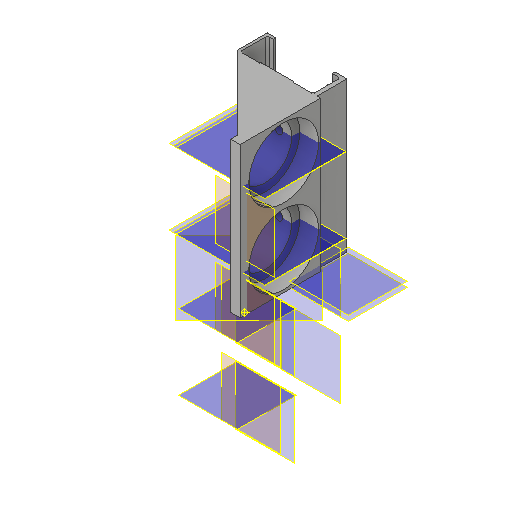
# Autodesk Inventor part: 30_Cube_Insert_Filter_Revolver_Filter_base_triple
Saved by Autodesk Inventor 2022 (Build 260153000, 153)
## iProperties
Created: 2021-09-13
Part Number: 30_Cube_Insert_Filter_Revolver_Filter_base_triple
Material: Generic
Document SubType Name: Modeling
Designer: diederichbenedict
Density: 1 g/cm^3
Appearance: Default
Mass: 6.97028 g
Surface Area: 48.8121 cm^2
Volume: 6.97028 cm^3
Author: diederichbenedict
Autodesk Inventor part; units mm, degrees
ref_plane "YZ Plane" through (0, 0, 0) normal (1, 0, 0) x (0, 1, 0)
ref_plane "XZ Plane" through (0, 0, 0) normal (0, 1, 0) x (-1, 0, 0)
ref_plane "XY Plane" through (0, 0, 0) normal (0, 0, 1) x (1, 0, 0)
ref_plane "Work Plane1" through (-34.3358, -34.38, 2.0699) normal (0, -1, 0) x (0.7071068, 0, -0.7071068)
ref_plane "Work Plane4" through (-9.5871, -34.38, 28.2329) normal (0, -1, 0) x (1, 0, 0)
ref_plane "Work Plane3" through (-9.5871, -32.38, 28.2329) normal (0, -1, 0) x (1, 0, 0)
sketch "Sketch1" plane through (-9.5871, -34.38, 28.2329) normal (0, -1, 0) x (1, 0, 0)
  line L0 (0.7071, -1.3185) -> (0.7071, -26.3185) construction
  line L1 (0.7071, -1.3185) -> (1.7071, -1.3185) construction
  line L2 (0.7071, -26.3185) -> (1.7071, -26.3185) construction
  line L3 (-4.2929, -0.7071) -> (-31.7929, -28.2071)
  line L4 (-31.7929, -28.2071) -> (0.7071, -28.2071)
  line L5 (0.7071, -28.2071) -> (0.7071, -0.7071)
  line L6 (0.7071, -0.7071) -> (-4.2929, -0.7071)
  line L7 (-4.2929, -0.7071) -> (-4.2929, -28.2071)
  line L8 (-4.2929, -28.2071) -> (0.7071, -28.2071)
  line L9 (0.7071, -0.7071) -> (3.5978, -0.7071)
  line L10 (2.5336, 1.8671) -> (2.3871, 1.8671) projected
  line L11 (0.7071, -0.7071) -> (0.7071, -28.2071)
  line L12 (0.7071, -28.2071) -> (-31.7929, -28.2071)
  point P0 (9.5871, -28.2329)
  dimension "d1" = 5
  dimension "d96" = 27.5
  dimension "d97" = 135
  constraints: 22 end point, 4 perpendicular, 3 horizontal, 2 point on line, 1 collinear, 2 other
  measures "d1" distance of L5.end L3.start
  measures "d96" distance between parallel lines of L4 L6
  measures "d97" angle of L7 L3
extrude "Extrusion1" add sketch "Sketch1" against normal blind 28
ref_plane "Work Plane5" through (-9.5871, -20.38, 28.2329) normal (0, -1, 0) x (1, 0, 0)
ref_plane "Work Plane6" through (-11.0013, -34.38, 27.5258) normal (0, 0, 1) x (1, 0, 0)
sketch "Sketch4" plane through (-8.88, -34.38, 27.5258) normal (-1, 0, 0) x (0, 0, 1)
  line L0 (0, 0) -> (-27.5, 0) projected
  line L1 (-27.5, 28) -> (0, 28) projected
  circle A0 centre (-13.75, 14) radius 10
  line L2 (0, 0) -> (0, 28) projected
  point P0 (-27.5258, 34.38)
  dimension "d89" = 28
  dimension "d90" = 20
  dimension "d91" = 14
  dimension "d98" = 13.75
  constraints: 1 centre point
  measures "d89" distance between parallel lines of L0 L1
  measures "d90" diameter of A0
  measures "d91" distance from line of A0.centre L0
  measures "d98" distance from line of A0.centre L2
extrude "Extrusion4" cut sketch "Sketch4" along normal through all
sketch "Sketch9" plane through (-11.38, -34.38, 30.0258) normal (-0.7071068, 0, 0.7071068) x (0.7071068, 0, 0.7071068)
  ellipse E0 centre (-22.981, 14) end of major axis (-37.1231, 14) minor radius 10 projected
  circle A0 centre (-22.981, 14) radius 13
  point P0 (-13.1846, 34.38)
  dimension "d129" = 26
  constraints: 1 centre point, 1 coincident, 1 other
  measures "d129" diameter of A0
extrude "Extrusion9" cut sketch "Sketch9" against normal blind 3.3 contours A0 E0 | E0 A0 | A0 E0 picked at (-32.6632, 13.9035) picked at (-21.8913, 2.1109) picked at (-24.0707, 25.8891)
sketch "Sketch3" plane through (-8.88, -34.38, 27.5258) normal (-1, 0, 0) x (0, 0, 1)
  circle A0 centre (-13.75, 14) radius 10 projected
  circle A1 centre (-13.75, 14) radius 13
  point P0 (-27.5258, 34.38)
  point P1 (13.1114, 14)
  dimension "d100" = 26
  constraints: 1 centre point, 1 coincident
  measures "d100" diameter of A1
extrude "Extrusion3" cut sketch "Sketch3" along normal blind 8.5 contours A0 | A1
sketch "Sketch13" plane through (-12.38, -34.38, 29.0258) normal (-0.7071068, 0, 0.7071068) x (0.7071068, 0, 0.7071068)
  arc A0 (-7.4246, 14) -> (-7.4246, 14) centre (-21.5668, 14) ccw projected
  circle A1 centre (-7.0668, 25) radius 1.4
  circle A2 centre (-7.0668, 3) radius 1.4
  circle A3 centre (-37.5668, 14) radius 1.4
  point P0 (-11.7703, 34.38)
  point P1 (-18.5424, 14)
  dimension "d101" = 2.8
  dimension "d102" = 2.8
  dimension "d103" = 14.5
  dimension "d104" = 14.5
  dimension "d105" = 16
  dimension "d106" = 2.8
  dimension "d127" = 11
  dimension "d128" = 11
  constraints: 3 centre point, 1 other
  measures "d101" diameter of A2
  measures "d102" diameter of A3
  measures "d103" horizontal distance of A1.centre point (-21.567, 14)
  measures "d104" horizontal distance of point (-21.567, 14) A2.centre
  measures "d105" distance of point (-21.567, 14) A3.centre
  measures "d106" diameter of A1
  measures "d127" vertical distance of A1.centre point (-21.567, 14)
  measures "d128" vertical distance of point (-21.567, 14) A2.centre
extrude "Extrusion13" cut sketch "Sketch13" against normal blind 10 contours A1 | A2 | A3
ref_plane "Arbeitsebene13" through (-3.6065, -62.7242, 27.5258) normal (0, 0, -1) x (-1, 0, 0)
ref_plane "Arbeitsebene16" through (-8.88, -62.38, 27.5258) normal (0, 0, 1) x (1, 0, 0)
sketch "Sketch16" plane through (-8.88, -62.38, 27.5258) normal (0, 0, 1) x (1, 0, 0)
  ellipse E0 centre (-13.3299, 42) end of major axis (-13.3299, 54.75) minor radius 9.0156 projected
  circle A0 centre (-13.3299, 42) radius 1.5708
  point P0 (8.88, 62.38)
  constraints: 1 centre point, 1 coincident, 1 other
extrude "Extrusion15" cut sketch "Sketch16" against normal through all contours A0
ref_plane "Work Plane11" through (-8.88, -20.38, 27.5258) normal (0, -1, 0) x (1, 0, 0)
ref_plane "Arbeitsebene12" through (-8.88, -20.38, 27.5258) normal (0, -1, 0) x (1, 0, 0)
ref_plane "Arbeitsebene15" through (-13.88, -62.38, 0.0258) normal (0, 0, -1) x (1, 0, 0)
sketch "Skizze20" plane through (-13.88, -62.38, 0.0258) normal (0, 0, -1) x (1, 0, 0)
  circle A0 centre (27.7649, 33.0797) radius 1.45
  point P0 (13.88, -62.38)
  dimension "d93" = 2.9
  constraints: 1 centre point
  measures "d93" diameter of A0
extrude "Extrusion17" cut sketch "Skizze20" against normal blind 10
ref_plane "Arbeitsebene14" through (-13.88, -62.38, 27.5258) normal (0, -1, 0) x (1, 0, 0)
sketch "Skizze22" plane through (-13.88, -34.38, 27.5258) normal (0, -1, 0) x (1, 0, 0)
  arc A0 (-18.7505, -36.1766) -> (-18.1728, -35.6773) centre (-19.2056, -35.0662) ccw projected
  arc A1 (-17.9795, -35.5555) -> (-18.1728, -35.6773) centre (-17.9577, -35.8046) ccw projected
  line L0 (-17.9795, -35.5555) -> (-17.6339, -35.5253) projected
  arc A2 (-17.6339, -35.5253) -> (-17.4056, -35.2762) centre (-17.6556, -35.2762) ccw projected
  line L1 (-17.4056, -35.2762) -> (-17.4056, -34.8238) projected
  arc A3 (-17.4056, -34.8238) -> (-17.6339, -34.5747) centre (-17.6556, -34.8238) ccw projected
  line L2 (-17.6339, -34.5747) -> (-18.0004, -34.5427) projected
  arc A4 (-18.1902, -34.4268) -> (-18.0004, -34.5427) centre (-17.9786, -34.2936) ccw projected
  arc A5 (-18.1902, -34.4268) -> (-18.7505, -33.9559) centre (-19.2056, -35.0662) ccw projected
  arc A6 (-18.9056, -33.7246) -> (-18.7505, -33.9559) centre (-18.6556, -33.7246) ccw projected
  line L3 (-18.9056, -33.7246) -> (-18.9056, -33.05) projected
  line L4 (-18.9056, -33.05) -> (-18.4056, -32.55) projected
  line L5 (-18.4056, -32.55) -> (-7.4056, -32.55) projected
  line L6 (-7.4056, -32.55) -> (-6.9056, -33.05) projected
  line L7 (-6.9056, -33.05) -> (-6.9056, -33.7246) projected
  arc A7 (-7.0608, -33.9559) -> (-6.9056, -33.7246) centre (-7.1556, -33.7246) ccw projected
  arc A8 (-7.0608, -33.9559) -> (-7.6211, -34.4268) centre (-6.6057, -35.0662) ccw projected
  arc A9 (-7.8109, -34.5427) -> (-7.6211, -34.4268) centre (-7.8327, -34.2936) ccw projected
  line L8 (-7.8109, -34.5427) -> (-8.1774, -34.5747) projected
  arc A10 (-8.1774, -34.5747) -> (-8.4056, -34.8238) centre (-8.1556, -34.8238) ccw projected
  line L9 (-8.4056, -34.8238) -> (-8.4056, -35.2762) projected
  arc A11 (-8.4056, -35.2762) -> (-8.1774, -35.5253) centre (-8.1556, -35.2762) ccw projected
  line L10 (-8.1774, -35.5253) -> (-7.8318, -35.5555) projected
  arc A12 (-7.6384, -35.6773) -> (-7.8318, -35.5555) centre (-7.8536, -35.8046) ccw projected
  arc A13 (-7.6384, -35.6773) -> (-7.0608, -36.1766) centre (-6.6057, -35.0662) ccw projected
  arc A14 (-6.9056, -36.4079) -> (-7.0608, -36.1766) centre (-7.1556, -36.4079) ccw projected
  line L11 (-6.9056, -36.4079) -> (-6.9056, -37.55) projected
  line L12 (-6.9056, -37.55) -> (-0.0057, -37.55) projected
  line L13 (-0.0057, -37.55) -> (0.5943, -36.95) projected
  line L14 (0.5943, -36.95) -> (0.5943, -33.55) projected
  arc A15 (0.5943, -32.75) -> (0.5943, -33.55) centre (0.8943, -33.15) ccw projected
  line L15 (0.5943, -32.75) -> (0.5943, -28.15) projected
  line L16 (0.5943, -28.15) -> (-0.0057, -27.55) projected
  line L17 (-0.0057, -27.55) -> (-6.5056, -27.55) projected
  line L18 (-6.5056, -27.55) -> (-6.9056, -27.95) projected
  line L19 (-6.9056, -27.95) -> (-18.9056, -27.95) projected
  line L20 (-18.9056, -27.95) -> (-19.3056, -27.55) projected
  line L21 (-19.3056, -27.55) -> (-25.8056, -27.55) projected
  line L22 (-25.8056, -27.55) -> (-26.4056, -28.15) projected
  line L23 (-26.4056, -28.15) -> (-26.4056, -36.95) projected
  line L24 (-26.4056, -36.95) -> (-25.8056, -37.55) projected
  line L25 (-25.8056, -37.55) -> (-18.9056, -37.55) projected
  line L26 (-18.9056, -37.55) -> (-18.9056, -36.4079) projected
  arc A16 (-18.7505, -36.1766) -> (-18.9056, -36.4079) centre (-18.6556, -36.4079) ccw projected
  line L27 (-26.5056, -28.1086) -> (-25.847, -27.45)
  line L28 (-25.847, -27.45) -> (-19.2642, -27.45)
  line L29 (-19.2642, -27.45) -> (-18.8642, -27.85)
  line L30 (-18.8642, -27.85) -> (-6.9471, -27.85)
  line L31 (-6.9471, -27.85) -> (-6.5471, -27.45)
  line L32 (-6.5471, -27.45) -> (0.0358, -27.45)
  line L33 (0.0358, -27.45) -> (0.6943, -28.1086)
  line L34 (0.6943, -28.1086) -> (0.6943, -32.8036)
  arc A17 (0.6943, -32.8036) -> (0.6943, -33.4964) centre (0.8943, -33.15) ccw
  line L35 (0.6943, -33.4964) -> (0.6943, -36.9914)
  line L36 (0.6943, -36.9914) -> (0.0358, -37.65)
  line L37 (0.0358, -37.65) -> (-7.0056, -37.65)
  line L38 (-7.0056, -37.65) -> (-7.0056, -36.4079)
  arc A18 (-7.0056, -36.4079) -> (-7.0988, -36.2691) centre (-7.1556, -36.4079) ccw
  arc A19 (-7.7245, -35.7282) -> (-7.0988, -36.2691) centre (-6.6057, -35.0662) ccw
  arc A20 (-7.7245, -35.7282) -> (-7.8405, -35.6551) centre (-7.8536, -35.8046) ccw
  line L39 (-7.8405, -35.6551) -> (-8.1862, -35.6249)
  arc A21 (-8.5056, -35.2762) -> (-8.1862, -35.6249) centre (-8.1556, -35.2762) ccw
  line L40 (-8.5056, -35.2762) -> (-8.5056, -34.8238)
  arc A22 (-8.1862, -34.4751) -> (-8.5056, -34.8238) centre (-8.1556, -34.8238) ccw
  line L41 (-8.1862, -34.4751) -> (-7.8196, -34.4431)
  arc A23 (-7.8196, -34.4431) -> (-7.7057, -34.3736) centre (-7.8327, -34.2936) ccw
  arc A24 (-7.0988, -33.8634) -> (-7.7057, -34.3736) centre (-6.6057, -35.0662) ccw
  arc A25 (-7.0988, -33.8634) -> (-7.0056, -33.7246) centre (-7.1556, -33.7246) ccw
  line L42 (-7.0056, -33.7246) -> (-7.0056, -33.0914)
  line L43 (-7.0056, -33.0914) -> (-7.4471, -32.65)
  line L44 (-7.4471, -32.65) -> (-18.3642, -32.65)
  line L45 (-18.3642, -32.65) -> (-18.8056, -33.0914)
  line L46 (-18.8056, -33.0914) -> (-18.8056, -33.7246)
  arc A26 (-18.8056, -33.7246) -> (-18.7125, -33.8634) centre (-18.6556, -33.7246) ccw
  arc A27 (-18.1056, -34.3736) -> (-18.7125, -33.8634) centre (-19.2056, -35.0662) ccw
  arc A28 (-18.1056, -34.3736) -> (-17.9917, -34.4431) centre (-17.9786, -34.2936) ccw
  line L47 (-17.9917, -34.4431) -> (-17.6251, -34.4751)
  arc A29 (-17.3056, -34.8238) -> (-17.6251, -34.4751) centre (-17.6556, -34.8238) ccw
  line L48 (-17.3056, -34.8238) -> (-17.3056, -35.2762)
  arc A30 (-17.6251, -35.6249) -> (-17.3056, -35.2762) centre (-17.6556, -35.2762) ccw
  line L49 (-17.6251, -35.6249) -> (-17.9708, -35.6551)
  arc A31 (-17.9708, -35.6551) -> (-18.0868, -35.7282) centre (-17.9577, -35.8046) ccw
  arc A32 (-18.7125, -36.2691) -> (-18.0868, -35.7282) centre (-19.2056, -35.0662) ccw
  arc A33 (-18.7125, -36.2691) -> (-18.8056, -36.4079) centre (-18.6556, -36.4079) ccw
  line L50 (-18.8056, -36.4079) -> (-18.8056, -37.65)
  line L51 (-18.8056, -37.65) -> (-25.8471, -37.65)
  line L52 (-25.8471, -37.65) -> (-26.5056, -36.9914)
  line L53 (-26.5056, -36.9914) -> (-26.5056, -28.1086)
  line L54 (-27.5, -27.5) -> (0, 0) projected
  line L55 (-27.5, -27.5) -> (-27.5, -38.65)
  line L56 (-27.5, -38.65) -> (-24.2729, -38.65)
  line L57 (-24.2729, -38.65) -> (-24.2729, -37.65)
  line L58 (5, -27.5) -> (5, 0) projected
  line L59 (5, 0) -> (0, 0) projected
  line L60 (0, 0) -> (-27.5, -27.5) projected
  line L61 (-27.5, -27.5) -> (5, -27.5) projected
  line L62 (5, 0) -> (5, -27.5) projected
  line L63 (2.1943, -38.65) -> (-2.2219, -38.65)
  line L64 (-2.2219, -38.65) -> (-2.2219, -37.65)
  line L65 (5, -27.5) -> (-27.5, -27.5) projected
  line L66 (2.1943, -38.65) -> (2.1943, -27.5)
  line L67 (5, -27.5) -> (5, -27.95)
  line L68 (5, -32.55) -> (5, -32.6858)
  point P0 (-18.4056, -35.2662)
  point P1 (-17.1577, -36.0046)
  point P2 (-16.8556, -35.4762)
  point P3 (-16.8556, -35.0238)
  point P4 (-17.1786, -34.4936)
  point P5 (-18.4056, -35.2662)
  point P6 (-17.8556, -33.9246)
  point P7 (-6.3556, -33.9246)
  point P8 (-5.8057, -35.2662)
  point P9 (-7.0327, -34.4936)
  point P10 (-7.3556, -35.0238)
  point P11 (-7.3556, -35.4762)
  point P12 (-7.0536, -36.0046)
  point P13 (-5.8057, -35.2662)
  point P14 (-6.3556, -36.6079)
  point P15 (1.6943, -33.35)
  point P16 (-17.8556, -36.6079)
  point P17 (5, -37.65)
  point P18 (-25.897, -27.5)
  point P19 (0.0857, -27.5)
  point P20 (0.0857, -27.5)
  point P21 (-6.5971, -27.5)
  point P22 (-19.2142, -27.5)
  point P23 (2.1943, -27.5)
  dimension "d133" = 0.1
  dimension "d134" = 1
  dimension "d135" = 1
  dimension "d141" = 1.5
  constraints: 70 end point, 34 point on circle, 17 centre point, 11 point on line, 4 perpendicular, 4 vertical, 1 parallel, 43 other
  measures "d133" distance between parallel lines of L22 L27
  measures "d134" distance between parallel lines of L51 L56
  measures "d135" distance between parallel lines of L37 L63
  measures "d141" distance between parallel lines of L66 L34
extrude "Extrusion18" add sketch "Skizze22" against normal up to surface (28 mm away) contours L53 L52 L51 L57 L56 L55 L61 L27 | L27 L28 L29 L61 | L61 L31 L30 L29 | L31 L32 L33 L61 | L61 L66 L63 L64 L37 L36 L35 A17 L34 L33
ref_plane "Arbeitsebene17" through (-13.88, -62.38, 27.5258) normal (0, -1, 0) x (1, 0, 0)
sketch "Skizze23" plane through (-13.88, -62.38, 27.5258) normal (0, -1, 0) x (1, 0, 0)
  line L0 (3, -39.05) -> (5, -37.05) projected
  line L1 (5.8412, 1.6556) -> (3.5, 1.6556)
  line L2 (3.5, 1.6556) -> (3.5, -38.55)
  line L3 (3.5, -38.55) -> (5.8412, -38.55)
  line L4 (5.8412, -38.55) -> (5.8412, 1.6556)
  line L5 (15.0143, 5.0596) -> (3, 5.0596)
  line L6 (3, 5.0596) -> (3, -44.8612)
  line L7 (3, -44.8612) -> (15.0143, -44.8612)
  line L8 (15.0143, -44.8612) -> (15.0143, 5.0596)
  point P0 (13.88, -27.5258)
  constraints: 16 end point, 4 parallel, 2 horizontal, 2 perpendicular, 1 point on line
extrude "Extrusion19" cut sketch "Skizze23" against normal through all contours L4 L3 L2 L1
sketch "Skizze24" plane through (-13.88, -34.38, 27.5258) normal (0, 0, 1) x (1, 0, 0)
  line L0 (3.5, 28) -> (5, 28) projected
  line L1 (3.5, 0) -> (3.5, 28) projected
  line L2 (5, 0) -> (3.5, 0) projected
  line L3 (5, 28) -> (5, 0) projected
  line L4 (3.5, 0) -> (3.5, 28) projected
  line L5 (0, 28) -> (3.5, 28) projected
  line L6 (0, 0) -> (0, 28) projected
  line L7 (3.5, 0) -> (0, 0) projected
  point P0 (13.88, 34.38)
extrude "Extrusion20" add sketch "Skizze24" along normal blind 2.5 contours L1 L7 L6 L5
pattern_linear "Rechteckige Anordnung4" count 2 spacing 28 along (0, 1, 0) of "Extrusion1", "Extrusion4", "Extrusion9", "Extrusion3", "Extrusion13", "Extrusion15", "Extrusion17", "Extrusion18", "Extrusion19", "Extrusion20"
ref_plane "Work Plane2" through (41.82, -7.88, -4) normal (0, -1, 0) x (1, 0, 0)
ref_plane "Arbeitsebene29" through (-11.0013, -6.38, 27.5258) normal (0, 0, 1) x (1, 0, 0)
ref_plane "Arbeitsebene30" through (-8.88, 7.62, 27.5258) normal (0, -1, 0) x (1, 0, 0)
ref_plane "Arbeitsebene31" through (-8.88, 7.62, 27.5258) normal (0, -1, 0) x (1, 0, 0)
ref_plane "Arbeitsebene32" through (-3.6065, -34.7242, 27.5258) normal (0, 0, -1) x (-1, 0, 0)
ref_plane "Arbeitsebene33" through (-13.88, -34.38, 27.5258) normal (0, -1, 0) x (1, 0, 0)
ref_plane "Arbeitsebene34" through (-13.88, -34.38, 0.0258) normal (0, 0, -1) x (1, 0, 0)
ref_plane "Arbeitsebene35" through (-8.88, -34.38, 27.5258) normal (0, 0, 1) x (1, 0, 0)
ref_plane "Arbeitsebene36" through (-13.88, -34.38, 27.5258) normal (0, -1, 0) x (1, 0, 0)
ref_plane "Arbeitsebene37" through (-9.5871, 7.62, 28.2329) normal (0, -1, 0) x (1, 0, 0)
equation "\"d91\" = 0.5 * d89"
equation "\"d98\" = 0.5 * d96"
body "Solid1"
